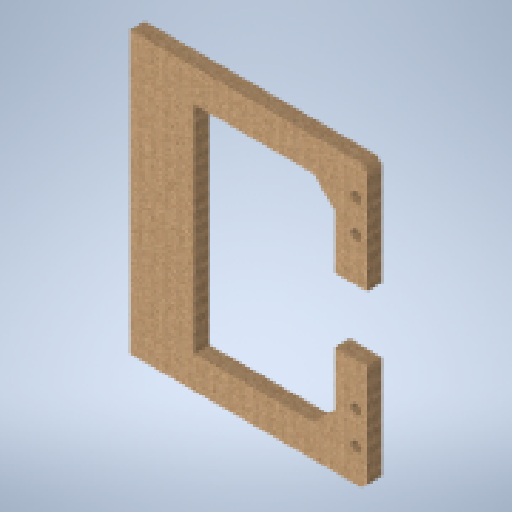
# Autodesk Inventor part: MarcoV2
Saved by Autodesk Inventor 2023.1 (Build 271208000, 208)
## iProperties
Created: 2022-10-30
Part Number: MarcoV2
Material: MDF Medium Density Fiberboard
Document SubType Name: Modeling
Designer: Daniel Peña
Density: 0.8 g/cm^3
Appearance: Cardboard - Corrugated
Author: Daniel Peña
Autodesk Inventor part; units mm, degrees
ref_plane "YZ Plane" through (0, 0, 0) normal (1, 0, 0) x (0, 1, 0)
ref_plane "XZ Plane" through (0, 0, 0) normal (0, 1, 0) x (-1, 0, 0)
ref_plane "XY Plane" through (0, 0, 0) normal (0, 0, 1) x (1, 0, 0)
sketch "Sketch1" plane through (0, 0, 0) normal (0, 0, 1) x (1, 0, 0)
  line L0 (-175, -7.5) -> (-230, -7.5)
  line L1 (-260, 7.5) -> (-152.5, 7.5)
  line L2 (-152.5, 7.5) -> (-150, 5)
  line L3 (-82.5, -57.5) -> (-255, -57.5)
  line L4 (-150, -42.5) -> (-165, -42.5)
  line L5 (-150, 5) -> (-150, -42.5)
  line L6 (-175, -7.5) -> (-165, -17.5)
  line L7 (-165, -42.5) -> (-165, -17.5)
  line L8 (-175, -107.5) -> (-230, -107.5)
  line L9 (-260, -122.5) -> (-152.5, -122.5)
  line L10 (-152.5, -122.5) -> (-150, -120)
  line L11 (-150, -72.5) -> (-165, -72.5)
  line L12 (-150, -120) -> (-150, -72.5)
  line L13 (-175, -107.5) -> (-165, -97.5)
  line L14 (-165, -72.5) -> (-165, -97.5)
  line L15 (-230, -7.5) -> (-230, -107.5)
  line L16 (-260, -122.5) -> (-260, 7.5)
  point P0 (0, 0)
  point P1 (-150, 7.5)
  dimension "d2" = -7.5
  dimension "d4" = 15
  dimension "d11" = 2.5
  dimension "d12" = 2.5
  dimension "d40" = 15
  dimension "d52" = 47.5
  dimension "d53" = 10
  dimension "d54" = 10
  dimension "d56" = 65
  dimension "d57" = 30
  constraints: 34 end point, 8 symmetric about line, 3 vertical, 2 horizontal
  measures "d2" distance from line of L0 point (0, 0)
  measures "d4" distance between parallel lines of L0 L1
  measures "d11" distance of L1.end point (-150, 7.5)
  measures "d12" distance of L2.end point (-150, 7.5)
  measures "d40" distance between parallel lines of L5 L7
  measures "d52" distance of L2.end L4.start
  measures "d53" horizontal distance of L0.start L6.end
  measures "d54" horizontal distance of L0.start L6.end
  measures "d56" distance between parallel lines of L15 L14
  measures "d57" distance between parallel lines of L16 L15
extrude "Extrusion1" add sketch "Sketch1" along normal blind 7
sketch "Sketch3" plane through (0, 0, 7) normal (0, 0, 1) x (1, 0, 0)
  line L0 (-155, 3.7259) -> (-155, -113.632) construction
  line L1 (-150, -42.5) -> (-150, 5) construction
  line L2 (-225, -107.5) -> (-225, -7.5) construction
  line L3 (-225, -57.375) -> (-3.3098, -57.375) construction
  point P0 (0, 0)
  point P1 (-155, -7.375)
  point P2 (-155, -22.375)
  point P3 (-155, -92.375)
  point P4 (-155, -107.375)
  point P5 (-230, -7.5)
  dimension "d41" = 5
  dimension "d42" = 15
  dimension "d43" = 70
  constraints: 4 end point, 4 point on line, 2 symmetric about line, 1 horizontal, 1 vertical, 2 other
  measures "d41" distance between parallel lines of L0 L1
  measures "d42" distance of point (-155, -92.375) point (-155, -107.375)
  measures "d43" distance of point (-155, -92.375) point (-155, -22.375)
hole "Hole2" at (-155, -7.375, 7) at (-155, -22.375, 7) at (-155, -92.375, 7) at (-155, -107.375, 7) direction (0, 0, -1) diameter 5 end through all
body "Solid1"
